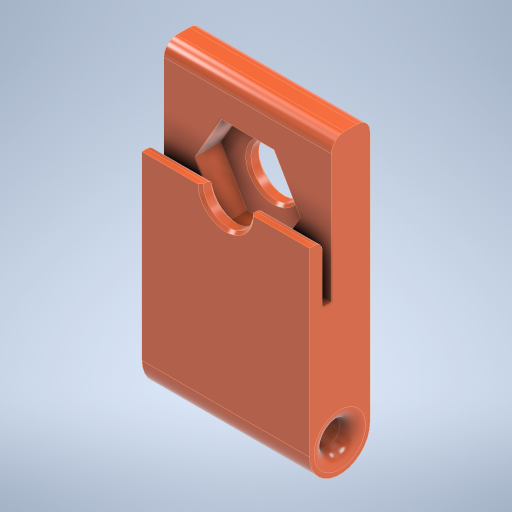
# Autodesk Inventor part: benniyebuçüklerinsiminibilmiyorum
Saved by Autodesk Inventor 2023.2 (Build 272271000, 271)
## iProperties
Created: 2022-11-27
Part Number: benniyebuçüklerinsiminibilmiyorum
Material: Generic
Document SubType Name: Modeling
Designer: omrfrkmll
Density: 1 g/cm^3
Appearance: Smooth - Light Orange
Author: omrfrkmll
Autodesk Inventor part; units mm, degrees
ref_plane "YZ Plane" through (0, 0, 0) normal (1, 0, 0) x (0, 1, 0)
ref_plane "XZ Plane" through (0, 0, 0) normal (0, 1, 0) x (-1, 0, 0)
ref_plane "XY Plane" through (0, 0, 0) normal (0, 0, 1) x (1, 0, 0)
sketch "Sketch1" plane through (0, 0, 0) normal (0, 0, 1) x (1, 0, 0)
  line L0 (0, 10.7195) -> (0, -8.2814)
  line L1 (-9.4164, 0) -> (11.224, 0)
  line L2 (-6.5, 6.5) -> (6.5, 6.5)
  line L3 (6.5, 6.5) -> (6.5, -6.5)
  line L4 (6.5, -6.5) -> (-6.5, -6.5)
  line L5 (-6.5, -6.5) -> (-6.5, 6.5)
  line L6 (-2.0496, 3.55) -> (2.0496, 3.55)
  line L7 (-2.0496, -3.55) -> (2.0496, -3.55)
  line L8 (-4.0992, 0) -> (-2.0496, 3.55)
  line L9 (2.0496, -3.55) -> (4.0992, 0)
  line L10 (-2.0496, -3.55) -> (-4.0992, 0)
  line L11 (4.0992, 0) -> (2.0496, 3.55)
  line L12 (2.0496, -3.55) -> (-2.0496, -3.55)
  line L13 (2.0496, 3.55) -> (-2.0496, 3.55)
  line L14 (4.0992, 0) -> (2.0496, -3.55)
  line L15 (-2.0496, 3.55) -> (-4.0992, 0)
  line L16 (2.0496, 3.55) -> (4.0992, 0)
  line L17 (-4.0992, 0) -> (-2.0496, -3.55)
  point P0 (0, 0)
  point P1 (4.0992, 0)
  dimension "d0" = 7.1
  dimension "d3" = 360
  dimension "d5" = 13
  dimension "d6" = 13
  constraints: 36 end point, 5 horizontal, 3 coincident, 2 parallel, 2 vertical, 1 perpendicular, 1 point on line, 40 other
  measures "d0" distance between parallel lines of L7 L6
  measures "d5" distance between parallel lines of L3 L5
  measures "d6" distance between parallel lines of L4 L2
extrude "Extrusion1" add sketch "Sketch1" along normal mid plane 2 contours L2 L3 L1 L11 L6 L0 | L0 L6 L8 L1 L5 L2 | L1 L10 L7 L0 L4 L5 | L3 L4 L0 L7 L9 L1
sketch "Sketch2" plane through (0, 0, -1) normal (0, 0, -1) x (-1, 0, 0)
  line L0 (6.5, -6.5) -> (-6.5, -6.5) projected
  line L1 (-6.5, 6.5) -> (6.5, 6.5)
  line L2 (6.5, 6.5) -> (6.5, -6.5)
  line L3 (6.5, -6.5) -> (-6.5, -6.5)
  line L4 (-6.5, -6.5) -> (-6.5, 6.5)
  circle A0 centre (0, 0) radius 1.95
  dimension "d11" = 3.9
  constraints: 8 end point, 2 parallel, 1 centre point, 1 coincident, 1 horizontal, 1 perpendicular
  measures "d11" diameter of A0
extrude "Extrusion2" add sketch "Sketch2" along normal blind 1
sketch "Sketch3" plane through (6.5, -6.5, 1) normal (1, 0, 0) x (0, 0, -1)
  line L0 (0, 13) -> (0, 0) projected
  line L1 (0, 2) -> (-0.7, 2)
  line L2 (-0.7, 2) -> (-0.7, 6.5)
  line L3 (-0.7, 6.5) -> (-1.7, 6.5)
  line L4 (-1.7, 6.5) -> (-1.7, 0)
  line L5 (-1.7, 0) -> (0, 0)
  line L6 (3, 0) -> (0, 0) projected
  line L7 (0, 0) -> (0, 2)
  point P0 (1, 6.5)
  dimension "d12" = 0.7
  dimension "d13" = 1
  dimension "d14" = 2
  constraints: 12 end point, 4 perpendicular, 2 point on line, 1 horizontal, 1 vertical
  measures "d12" distance between parallel lines of L0 L2
  measures "d13" distance between parallel lines of L2 L4
  measures "d14" distance between parallel lines of L5 L1
extrude "Extrusion3" add sketch "Sketch3" against normal up to surface (13 mm away)
sketch "Sketch4" plane through (6.5, -6.5, 2.7) normal (0, 0, 1) x (1, 0, 0)
  circle A0 centre (-6.5, 6.5) radius 1.95
  dimension "d17" = 3.9
  constraints: 1 centre point, 1 coincident
  measures "d17" diameter of A0
extrude "Extrusion4" cut sketch "Sketch4" against normal through all
chamfer "Chamfer1" distance 0.2 angle 45 4 edges at (0, -1.95, 2.7) (0, -1.95, 1.7) (1.95, 0, -1) (1.95, 0, -2)
sketch "Sketch5" plane through (6.5, -6.5, -2) normal (1, 0, 0) x (0, 0, -1)
  line L0 (-2.35, -2.8361) -> (-2.35, 14.8479)
  circle A0 centre (-2.35, -7.5322) radius 1
  line L1 (0, 0) -> (0, -7.5322)
  line L2 (0, 0) -> (-4.7, 0) projected
  line L3 (-4.7, -7.5322) -> (-4.7, 0)
  arc A1 (-4.7, -7.5322) -> (0, -7.5322) centre (-2.35, -7.5322) ccw
  point P0 (-2, 6.5)
  dimension "d23" = 2
  dimension "d26" = 7.5322
  constraints: 6 end point, 3 vertical, 2 centre point, 2 point on circle, 1 point on line, 1 tangent
  measures "d23" diameter of A0
  measures "d26" distance from line of L2 A0.centre
extrude "Extrusion5" add sketch "Sketch5" against normal up to surface (13 mm away)
fillet "Fillet1" radius 0.6 2 edges at (4.325, 0, 1.7) (-4.325, 0, 1.7)
fillet "Fillet2" radius 1 2 edges at (6.5, -14.0322, 1.35) (-6.5, -14.0322, 1.35)
fillet "Fillet3" radius 1 2 edges at (0, 6.5, -2) (0, 6.5, 1)
body "Solid1"
